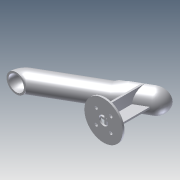
# Autodesk Inventor part: carousel_mount_rev4
Saved by Autodesk Inventor 2011 (Build 150239000, 239)
## iProperties
Created: 2012-11-18
Part Number: carousel_mount_rev4
Document SubType Name: Modeling
Designer: Administrator
Density: 1 g/cm^3
Author: Administrator
Autodesk Inventor part; units mm, degrees
ref_plane "YZ Plane" through (0, 0, 0) normal (1, 0, 0) x (0, 1, 0)
ref_plane "XZ Plane" through (0, 0, 0) normal (0, 1, 0) x (-1, 0, 0)
ref_plane "XY Plane" through (0, 0, 0) normal (0, 0, 1) x (1, 0, 0)
sketch "Skelethon sketch" plane through (0, 0, 0) normal (0, 0, 1) x (1, 0, 0)
  line L0 (0, 0) -> (45, 25.9808) construction
  line L1 (45, 25.9808) -> (45, 0) construction
  line L2 (45, 0) -> (0, 0) construction
  line L3 (0, 0) -> (0, -11) construction
  line L4 (0, 0) -> (-19.0526, -11) construction
  line L5 (45, 25.9808) -> (57.9904, 33.4808) construction
  dimension "d0" = 30
  dimension "d1" = 45
  dimension "d13" = 11
  dimension "d17" = 15
  constraints: 12 end point, 2 collinear, 2 perpendicular, 1 horizontal alignment, 1 vertical
  measures "d0" angle of L2 L0
  measures "d1" distance of L1.end L0.start
  measures "d13" distance of L0.start L3.end
  measures "d17" distance of L0.end L5.end
sketch "Sketch2" plane through (0, 0, 0) normal (0, 1, 0) x (-1, 0, 0)
  circle A0 centre (-45, 0) radius 18.5
  circle A1 centre (-45, 0) radius 4.5
  line L0 (-45, 0) -> (-45, 18.5) construction
  line L1 (-45, 0) -> (-58.0815, 13.0815) construction
  circle A2 centre (-52.0711, 7.0711) radius 1.5
  circle A3 centre (-52.0711, -7.0711) radius 1.5
  circle A4 centre (-37.9289, -7.0711) radius 1.5
  circle A5 centre (-37.9289, 7.0711) radius 1.5
  point P0 (0, 0)
  dimension "d2" = 37
  dimension "d3" = 9
  dimension "d4" = 45
  dimension "d5" = 10
  dimension "d6" = 3
  dimension "d9" = 360
  constraints: 6 centre point, 4 end point, 2 coincident, 2 point on circle, 1 point on line, 1 vertical, 9 other
  measures "d2" diameter of A0
  measures "d3" diameter of A1
  measures "d4" angle of L0 L1
  measures "d5" distance of point (-45, 0) A2.centre
  measures "d6" diameter of A2
extrude "wheel extr" add sketch "Sketch2" along normal blind 1.75
ref_plane "Tube Ref plane" through (-19.0526, -11, 0) normal (-0.8660254, -0.5, 0) x (0.5, -0.8660254, 0)
ref_plane "Tube ut_Ref Plane" through (45, 25.9808, 0) normal (0.8660254, 0.5, 0) x (-0.5, 0.8660254, 0)
ref_plane "Tube ut_ProfileRef Plane" through (57.9904, 33.4808, 0) normal (0.8660254, 0.5, 0) x (-0.5, 0.8660254, 0)
ref_plane "Tube ut_profileRef Plane2" through (41.7524, 24.1058, 0) normal (0.8660254, 0.5, 0) x (-0.5, 0.8660254, 0)
sketch "Sketch4" plane through (-19.0526, -11, 0) normal (-0.8660254, -0.5, 0) x (0.5, -0.8660254, 0)
  circle A0 centre (-9.25, 0) radius 9.25
  line L0 (-9.25, 0) -> (0, 0) construction
  circle A1 centre (-9.25, 0) radius 7.5 construction
  dimension "d20" = 1.75
  dimension "d67" = 15
  constraints: 2 coincident, 2 end point, 2 horizontal alignment, 1 centre point, 2 other
  measures "d67" diameter of A1
ref_plane "Tube ut_profileRef Plane3" through (32.0096, 18.4808, 0) normal (0.8660254, 0.5, 0) x (-0.5, 0.8660254, 0)
sketch "Sketch6" plane through (32.0096, 18.4808, 0) normal (0.8660254, 0.5, 0) x (-0.5, 0.8660254, 0)
  circle A0 centre (9.25, 0) radius 9.25 projected
  circle A1 centre (9.25, 0) radius 7.5 projected
  point P0 (0, 0)
  constraints: 1 horizontal alignment
sketch "Sketch7" plane through (41.7524, 24.1058, 0) normal (0.8660254, 0.5, 0) x (-0.5, 0.8660254, 0)
  circle A0 centre (11.875, 0) radius 10.125
  circle A1 centre (11.875, 0) radius 11.875
  line L0 (11.875, 0) -> (0, 0) construction
  dimension "d22" = 20.25
  dimension "d23" = 1.75
  constraints: 2 coincident, 2 end point, 1 centre point, 1 horizontal, 1 horizontal alignment, 2 other
  measures "d22" diameter of A0
sketch "Sketch8" plane through (57.9904, 33.4808, 0) normal (0.8660254, 0.5, 0) x (-0.5, 0.8660254, 0)
  circle A0 centre (11.875, 0) radius 11.875 projected
  circle A1 centre (11.875, 0) radius 10.125 projected
  point P0 (0, 0)
  constraints: 1 horizontal alignment
loft "middle loft transition" add profiles "Sketch6", "Sketch7" contours A0 | A1 / A0 | A1
loft "middle loft transcut" cut profiles "Sketch6", "Sketch7" contours A1 / A0
sketch "Sketch10" plane through (35.8149, 34.3898, 0) normal (0.8660254, 0.5, 0) x (0, 0, -1)
  circle A0 centre (0, 0) radius 10.125 projected
  circle A1 centre (0, 0) radius 11.875 projected
  line L0 (0, 11.875) -> (0, 11.875) construction
  point P0 (0, -11.875)
  constraints: 2 end point, 2 point on circle, 1 horizontal, 1 tangent
extrude "catch tube solid" add sketch "Sketch10" along normal up to surface (18.75 mm away)
sketch "Sketch11" plane through (27.3846, 26.4915, 0) normal (-0.8660254, -0.5, 0) x (0, 0, 1)
  circle A0 centre (0, 0) radius 7.5 projected
  circle A1 centre (0, 0) radius 9.25 projected
  point P0 (0, -9.25)
  constraints: 1 vertical alignment
extrude "exit tube solid" add sketch "Sketch11" along normal up to surface (58.9615 mm away)
sketch "cut height ref sketch" plane through (52.0529, 43.7648, 0) normal (0.8660254, 0.5, 0) x (0, 0, -1)
  circle A0 centre (0, 0) radius 10.125 projected
  circle A1 centre (0, 0) radius 11.875 projected
  line L0 (-11.8328, -1) -> (11.8328, -1) construction
  line L1 (0, 11.875) -> (0, 11.875) construction
  line L2 (-10.125, 0) -> (-11.875, 0)
  line L3 (10.125, 0) -> (11.875, 0)
  line L4 (-10.125, 0) -> (10.125, 0)
  point P0 (0, -11.875)
  dimension "d42" = 10.875
  constraints: 10 end point, 2 collinear, 2 horizontal, 2 parallel, 2 point on circle, 2 point on line, 7 other
  measures "d42" distance from line of point (0, -11.875) L0
sketch "Sketch13" plane through (0, 0, 0) normal (0, 0, 1) x (1, 0, 0)
  line L0 (32.0096, 18.4808) -> (22.7596, 34.5022) construction
  line L1 (30.7524, 43.1583) -> (40.8774, 25.6213) construction
  line L2 (29.8774, 44.6739) -> (46.1154, 54.0489) construction
  line L3 (52.5529, 42.8988) -> (36.3149, 33.5238)
  arc A0 (22.7596, 34.5022) -> (36.3149, 33.5238) centre (30.2591, 44.0128) ccw
  line L4 (22.7596, 34.5022) -> (11.5721, 53.8796)
  line L5 (57.1154, 34.9963) -> (46.9904, 52.5333) projected
  line L6 (52.5529, 42.8988) -> (37.5529, 68.8796)
  line L7 (11.5721, 53.8796) -> (37.5529, 68.8796)
  point P0 (0, 0)
  dimension "d80" = 30
  constraints: 8 end point, 2 parallel, 2 perpendicular, 2 point on circle, 1 centre point, 1 coincident, 1 point on line, 1 tangent
  measures "d80" distance of L3.start L6.end
extrude "catch tube solid cut" cut sketch "Sketch13" along normal through all both and the other way through all
sketch "Sketch14" plane through (45, 1.75, 0) normal (0, 1, 0) x (1, 0, 0)
  circle A0 centre (0, 0) radius 18.5 projected
  line L0 (0, 0) -> (0, 18.5) construction
  line L1 (0, 0) -> (18.5, 0) construction
  line L2 (7.5529, 11.8328) -> (0, 11.8328) construction
  line L3 (0, 0) -> (0, -18.5) construction
  line L4 (7.5529, -11.8328) -> (0, -11.8328) construction
  line L5 (-0.875, 11.8328) -> (0.875, 11.8328)
  line L6 (0.875, 11.8328) -> (0.875, -11.8328)
  line L7 (0.875, -11.8328) -> (-0.875, -11.8328)
  line L8 (-0.875, -11.8328) -> (-0.875, 11.8328)
  line L9 (-11.8328, 0.875) -> (11.8328, 0.875)
  line L10 (11.8328, 0.875) -> (11.8328, -0.875)
  line L11 (11.8328, -0.875) -> (-11.8328, -0.875)
  line L12 (-11.8328, -0.875) -> (-11.8328, 0.875)
  point P0 (-45, 0)
  point P1 (0, 0.875)
  dimension "d46" = 1.75
  constraints: 26 end point, 7 perpendicular, 5 parallel, 3 midpoint, 3 point on circle, 2 horizontal, 2 point on line, 1 vertical, 1 vertical alignment, 2 other
  measures "d46" distance between parallel lines of L8 L6
extrude "tube support" add sketch "Sketch14" along normal up to next contours L5 L6 L9 L8 | L9 L6 L11 L8 | L8 L11 L12 L9 | L9 L10 L11 L6 | L11 L6 L7 L8
sketch "exit endcap top" plane through (0, 0, 0) normal (0, 0, 1) x (1, 0, 0)
  line L0 (-19.0526, -11) -> (-28.3026, 5.0215) projected
  point P0 (0, 0)
ref_plane "exit  endcap plane" through (-19.0526, -11, 0) normal (0, 1, 0) x (-1, 0, 0)
sketch "exit encap sketch" plane through (-19.0526, -11, 0) normal (0, 1, 0) x (-1, 0, 0)
  circle A0 centre (9.25, 0) radius 9.25
  circle A1 centre (9.25, 0) radius 7.5
  line L0 (0, 0) -> (9.25, 0) construction
  point P0 (-19.0526, 0)
  dimension "d65" = 1.75
  dimension "d66" = 15
  constraints: 2 coincident, 2 end point, 1 centre point, 1 horizontal, 1 horizontal alignment, 2 other
  measures "d66" diameter of A1
sketch "Sketch33" plane through (0, 0, 0) normal (0, 0, 1) x (1, 0, 0)
  line L0 (-19.0526, -11) -> (-28.3026, 5.0215) projected
  line L1 (-19.0526, -11) -> (-37.5526, -11) projected
  arc A0 (-23.6776, -2.9893) -> (-28.3026, -11) centre (-19.0526, -11) ccw
  point P0 (0, 0)
  constraints: 2 point on circle, 1 centre point, 1 coincident
sweep "exit encap" add profiles "exit encap sketch" path "Sketch33" path curves A0
ref_plane "catch tube open plane" through (45, 38.5381, -11.8328) normal (-0.5, 0.8660254, 0) x (0.8660254, 0.5, 0)
revolve "top endcap" add sketch "cut height ref sketch" angle 180 about axis through (52.0529, 43.7648, 10.125) along (0, 0, 1) picked at (11.1766, -0.9473) contours L3 A1 L2 A0
sketch "Sketch32" plane through (0, 0, 0) normal (0, 0, 1) x (1, 0, 0)
  line L0 (52.5529, 42.8988) -> (46.1154, 54.0489) projected
  line L1 (52.5529, 42.8988) -> (37.5529, 68.8796)
  line L2 (37.5529, 68.8796) -> (63.5336, 83.8796)
  line L3 (63.5336, 83.8796) -> (78.5336, 57.8988)
  line L4 (78.5336, 57.8988) -> (52.5529, 42.8988)
  point P0 (0, 0)
  dimension "d76" = 30
  constraints: 8 end point, 4 perpendicular, 1 collinear
  measures "d76" distance between parallel lines of L4 L2
extrude "top endcap cut" cut sketch "Sketch32" along normal mid plane 30
ref_plane "exit tube checking plane" through (22.7596, 34.5022, 0) normal (-0.5, 0.8660254, 0) x (-0.8660254, -0.5, 0)
sketch "Sketch34" plane through (22.7596, 34.5022, 0) normal (-0.5, 0.8660254, 0) x (-0.8660254, -0.5, 0)
  line L0 (5, 1.75) -> (58.9615, 1.75)
  line L1 (58.9615, 1.75) -> (58.9615, -1.75)
  line L2 (58.9615, -1.75) -> (5, -1.75)
  line L3 (5, -1.75) -> (5, 1.75)
  line L4 (0, 7.5) -> (0, -7.5) projected
  line L5 (58.9615, -7.5) -> (58.9615, 7.5) projected
  point P0 (36.9615, 0)
  point P1 (58.9615, 0)
  point P2 (58.9615, 0)
  dimension "d82" = 5
  dimension "d83" = 0
  dimension "d86" = 3.5
  constraints: 8 end point, 2 midpoint, 2 parallel, 1 coincident, 1 horizontal, 1 perpendicular
  measures "d82" distance between parallel lines of L3 L4
  measures "d83" distance between parallel lines of L5 L1
  measures "d86" distance between parallel lines of L2 L0
extrude "exit tube checking cut" cut sketch "Sketch34" against normal up to surface round surface about axis through (27.3846, 26.4915, 0) along (-0.8660254, -0.5, 0) radius 7.5 far side no
equation "\"d0\" = angel"
equation "\"d1\" = exit_tube_length"
equation "\"d13\" = exit_tube_servo_offset"
equation "\"d17\" = catch_distance_tube"
equation "\"d3\" = circle_hole"
equation "\"d6\" = screw_mounting_hole"
equation "\"d11\" = wall_thickness"
equation "\"d20\" = wall_thickness"
equation "\"d67\" = tube_ID"
equation "\"d22\" = catch_tube_ID"
equation "\"d23\" = wall_thickness"
equation "\"d42\" = catch_tube_cut_height"
equation "\"d46\" = wall_thickness"
equation "\"d65\" = wall_thickness"
equation "\"d66\" = tube_ID"
equation "\"angel\" = 30deg"
equation "\"exit_tube_length\" = 45"
equation "\"wall_thickness\" = 1.75"
equation "\"wheel_diameter\" = 37"
equation "\"circle_hole\" = 9"
equation "\"screw_mounting_hole\" = 3"
equation "\"catch_distance_tube\" = 15"
equation "\"tube_ID\" = 15"
equation "\"d19\" = -0.25 * catch_distance_tube"
equation "\"d21\" = -0.75 * catch_distance_tube"
equation "\"catch_tube_ID\" = tube_ID + 3 * wall_thickness"
equation "\"exit_tube_servo_offset\" = 11"
equation "\"catch_tube_cut_height\" = 10.875"
body "Solid1"
